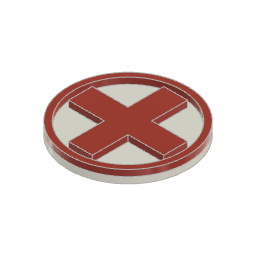
_4 Way.8ba9eb2e-5a56-47aa-8705-fbdcbb0d557d (Autodesk Fusion 360 design; units mm, degrees)
Autodesk Fusion 360 part; units mm, degrees
sketch "Sketch1" plane through (0, 0, 0) normal (0, 0, 1) x (1, 0, 0)
  circle A0 centre (0, 0) radius 15.875
  circle A1 centre (0, 0) radius 14.2875
  line L0 (0, 12.7) -> (3.175, 12.7)
  line L1 (3.175, 12.7) -> (3.175, 0)
  line L2 (3.175, 0) -> (0, 0)
  line L3 (0, 0) -> (0, 12.7)
  line L4 (0, 0) -> (3.175, 0)
  line L5 (3.175, 0) -> (3.175, -12.7)
  line L6 (3.175, -12.7) -> (0, -12.7)
  line L7 (0, -12.7) -> (0, 0)
  line L8 (0, -12.7) -> (-3.175, -12.7)
  line L9 (-3.175, -12.7) -> (-3.175, 12.7)
  line L10 (-3.175, 12.7) -> (0, 12.7)
  line L11 (0, 12.7) -> (0, -12.7)
  line L12 (0, 0) -> (12.7, 0)
  line L13 (12.7, 0) -> (12.7, 3.175)
  line L14 (12.7, 3.175) -> (0, 3.175)
  line L15 (0, 3.175) -> (0, 0)
  line L16 (0, 0) -> (12.7, 0)
  line L17 (12.7, 0) -> (12.7, -3.175)
  line L18 (12.7, -3.175) -> (0, -3.175)
  line L19 (0, -3.175) -> (0, 0)
  line L20 (0, 3.175) -> (-12.7, 3.175)
  line L21 (-12.7, 3.175) -> (-12.7, -3.175)
  line L22 (-12.7, -3.175) -> (0, -3.175)
  line L23 (0, -3.175) -> (0, 3.175)
  dimension "d1" = 31.75
  dimension "d2" = 28.575
  dimension "d3" = 3.175
  dimension "d4" = 12.7
  dimension "d5" = 3.175
  dimension "d6" = 12.7
  dimension "d7" = 3.175
  dimension "d8" = 3.175
  dimension "d9" = 12.7
  constraint coincident A0.centre A1.centre
  constraint concentric A0 A1
  constraint horizontal L0
  constraint vertical L1
  constraint horizontal L2
  constraint vertical L3
  constraint horizontal L4
  constraint vertical L5
  constraint horizontal L6
  constraint vertical L7
  constraint horizontal L8
  constraint vertical L9
  constraint horizontal L10
  constraint vertical L11
  constraint horizontal L12
  constraint vertical L13
  constraint horizontal L14
  constraint vertical L15
  constraint horizontal L16
  constraint vertical L17
  constraint horizontal L18
  constraint vertical L19
  constraint horizontal L20
  constraint vertical L21
  constraint horizontal L22
  constraint vertical L23
  measures "d1" diameter of A0
  measures "d2" diameter of A1
  measures "d3" distance of L0.start L0.end
  measures "d4" distance of A0.centre L6.end
  measures "d5" distance of L6.end L8.end
  measures "d6" distance of A0.centre L12.end
  measures "d7" distance of A0.centre L14.end
  measures "d8" distance of A0.centre L18.end
  measures "d9" distance of L14.end L20.end
extrude "Extrude1" add sketch "Sketch1" against normal blind 1 contours A0 | A1 | L0 L1 L3 L11 L14 | L3 L9 L10 L11 L20 | L1 L2 L3 L4 L11 L12 L14 L15 L16 L23 | L3 L7 L9 L11 L15 L19 L20 L22 L23 | L1 L12 L13 L14 L16 | L2 L4 L5 L7 L11 L12 L16 L18 L19 L23 | L9 L20 L21 L22 | L5 L12 L16 L17 L18 | L5 L6 L7 L11 L18 | L7 L8 L9 L11 L22 makes body 1 in component "Base"
extrude "Extrude1'" add sketch "Sketch1" along normal blind 1 separate body makes body 2 at (1.0583, 6.35, 0) makes body 3 at (15.2335, -1.4985, 0) in component "Top"
scale "Scale1" factors (0.6, 0.6, 1) about (-3.175, 3.175, 0) bodies 1 in component "Base"
scale "Scale1'" factors (0.6, 0.6, 1) about (-3.175, 3.175, 0) bodies 2 3 in component "Top"
component "Base" placed x (1, 0, 0) y (0, 1, 0) z (0, 0, 1) at (0, 0, 0)
component "Top" placed x (1, 0, 0) y (0, 1, 0) z (0, 0, 1) at (0, 0, 0)
